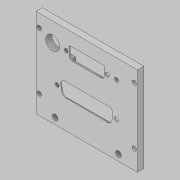
# Autodesk Inventor part: Rückwand_DVI
Saved by Autodesk Inventor 2021.4 (Build 254397000, 397)
## iProperties
Created: 2019-10-17
Part Number: Rückwand_DVI
Material: Generisch
Document SubType Name: Modeling
Designer: Scope
Density: 1 g/cm^3
Appearance: Vorgabe
Author: Scope
Autodesk Inventor part; units mm, degrees
ref_plane "YZ Plane" through (0, 0, 0) normal (1, 0, 0) x (0, 1, 0)
ref_plane "XZ Plane" through (0, 0, 0) normal (0, 1, 0) x (-1, 0, 0)
ref_plane "XY Plane" through (0, 0, 0) normal (0, 0, 1) x (1, 0, 0)
sketch "Skizze1" plane through (0, 0, 0) normal (0, 0, 1) x (1, 0, 0)
  line L0 (-40, 35) -> (40, 35)
  line L1 (40, 35) -> (40, -35)
  line L2 (40, -35) -> (-40, -35)
  line L3 (-40, -35) -> (-40, 35)
  line L4 (-40, 35) -> (40, -35) construction
  line L5 (40, 35) -> (-40, -35) construction
  point P0 (0, 0)
  dimension "d0" = 80
  dimension "d1" = 70
  constraints: 12 end point, 2 midpoint, 2 parallel, 1 horizontal, 1 perpendicular
  measures "d0" distance between parallel lines of L1 L3
  measures "d1" distance between parallel lines of L2 L0
extrude "Extrusion1" add sketch "Skizze1" along normal blind 5
sketch "Skizze2" plane through (0, 0, 5) normal (0, 0, 1) x (1, 0, 0)
  line L0 (-37.5, 25) -> (37.5, 25)
  line L1 (37.5, 25) -> (37.5, -20)
  line L2 (37.5, -20) -> (-37.5, -20)
  line L3 (-37.5, -20) -> (-37.5, 25)
  line L4 (-40, 35) -> (-40, -35) projected
  line L5 (40, -35) -> (40, 35) projected
  line L6 (-40, -35) -> (40, -35) projected
  point P0 (0, 0)
  dimension "d4" = 2.5
  dimension "d5" = 2.5
  dimension "d6" = 15
  dimension "d7" = 60
  constraints: 8 end point, 2 parallel, 1 horizontal, 1 perpendicular
  measures "d4" distance between parallel lines of L3 L4
  measures "d5" distance between parallel lines of L5 L1
  measures "d6" distance between parallel lines of L2 L6
  measures "d7" distance between parallel lines of L0 L6
hole "Bohrung1" at (-37.5, 25, 5) at (37.5, 25, 5) at (37.5, -20, 5) at (-37.5, -20, 5) direction (0, 0, -1) diameter 3.4 end through all clearance for "Flachkopfmaschinenschraube" size "M3" standard "ANSI Metrisches M Profil"
sketch "Skizze3" plane through (0, 0, 5) normal (0, 0, 1) x (1, 0, 0)
  line L0 (-25, -30) -> (25, -30)
  line L1 (-40, 35) -> (-40, -35) projected
  line L2 (40, -35) -> (40, 35) projected
  line L3 (-40, -35) -> (40, -35) projected
  point P0 (0, 0)
  dimension "d15" = 15
  dimension "d16" = 15
  dimension "d17" = 5
  constraints: 2 end point, 1 horizontal
  measures "d15" distance from line of L1 L0.start
  measures "d16" distance from line of L0.end L2
  measures "d17" distance between parallel lines of L3 L0
hole "Bohrung2" at (-25, -30, 5) at (25, -30, 5) direction (0, 0, -1) diameter 4.5 end through all clearance for "Flachkopfmaschinenschraube" size "M4" standard "ANSI Metrisches M Profil"
sketch "Skizze4" plane through (0, 0, 5) normal (0, 0, 1) x (1, 0, 0)
  line L0 (-13.15, 24.8) -> (13.15, 24.8)
  line L1 (13.75, 24.2) -> (13.75, 17.7)
  line L2 (11.25, 15.2) -> (-11.25, 15.2)
  line L3 (-13.75, 17.7) -> (-13.75, 24.2)
  line L4 (-13.75, 24.8) -> (13.75, 15.2) construction
  line L5 (13.75, 24.8) -> (-13.75, 15.2) construction
  line L6 (40, 35) -> (-40, 35) projected
  arc A0 (-13.15, 24.8) -> (-13.75, 24.2) centre (-13.15, 24.2) ccw
  arc A1 (13.75, 24.2) -> (13.15, 24.8) centre (13.15, 24.2) ccw
  arc A2 (-13.75, 17.7) -> (-11.25, 15.2) centre (-11.25, 17.7) ccw
  arc A3 (11.25, 15.2) -> (13.75, 17.7) centre (11.25, 17.7) ccw
  line L7 (48.751, 18.7264) -> (89.4803, 18.7264) construction
  line L8 (89.4803, 18.7264) -> (89.4803, 14.9967) construction
  line L9 (89.4803, 14.9967) -> (48.751, 14.9967) construction
  line L10 (48.751, 14.9967) -> (48.751, 18.7264) construction
  line L11 (-17.198, -1.3) -> (17.198, -1.3)
  line L12 (21.25, -1.3) -> (21.25, -1.3)
  line L13 (16.3869, -12.7) -> (-16.3869, -12.7)
  line L14 (-21.25, -1.3) -> (-21.25, -1.3)
  line L15 (-21.25, -1.3) -> (21.25, -12.7) construction
  line L16 (21.25, -1.3) -> (-21.25, -12.7) construction
  line L17 (-40, -35) -> (40, -35) projected
  line L18 (-20.5464, -5.2904) -> (-19.7353, -9.8904)
  line L19 (20.5464, -5.2904) -> (19.7353, -9.8904)
  arc A4 (-17.198, -1.3) -> (-20.5464, -5.2904) centre (-17.198, -4.7) ccw
  arc A5 (20.5464, -5.2904) -> (17.198, -1.3) centre (17.198, -4.7) ccw
  arc A6 (-19.7353, -9.8904) -> (-16.3869, -12.7) centre (-16.3869, -9.3) ccw
  arc A7 (16.3869, -12.7) -> (19.7353, -9.8904) centre (16.3869, -9.3) ccw
  line L20 (50.079, -7.9738) -> (119.9486, -7.9738) construction
  line L21 (119.9486, -7.9738) -> (119.9486, -12.597) construction
  line L22 (119.9486, -12.597) -> (50.079, -12.597) construction
  line L23 (50.079, -12.597) -> (50.079, -7.9738) construction
  line L24 (40, -35) -> (40, 35) projected
  point P0 (0, 0)
  point P1 (0, 20)
  point P2 (0, 20)
  point P3 (0, -7)
  point P4 (0, -7)
  point P5 (0, -7)
  point P6 (-19.2399, -12.7)
  point P7 (19.2399, -12.7)
  dimension "d25" = 27.5
  dimension "d26" = 9.6
  dimension "d28" = 0.6
  dimension "d29" = 2.5
  dimension "d32" = 15
  dimension "d49" = 28
  dimension "d50" = 11.4
  dimension "d51" = 42.5
  dimension "d52" = 80
  dimension "d53" = 19.2399
  dimension "d54" = 19.2399
  dimension "d55" = 80
  dimension "d56" = 3.4
  dimension "d64" = 26.25
  constraints: 28 end point, 20 point on line, 16 point on circle, 16 tangent, 8 centre point, 7 midpoint, 5 equal radius, 4 parallel, 2 horizontal, 2 perpendicular, 2 vertical alignment, 4 other
  measures "d25" distance between parallel lines of L1 L3
  measures "d26" distance of L5.start L4.end
  measures "d28" radius of A0
  measures "d29" radius of A2
  measures "d32" distance from line of L6 point (0, 20)
  measures "d49" distance from line of L17 point (0, -7)
  measures "d50" distance between parallel lines of L13 L11
  measures "d51" distance between parallel lines of L12 L14
  measures "d52" angle of L11 L18
  measures "d53" horizontal distance of point (0, -7) point (-19.24, -12.7)
  measures "d54" horizontal distance of point (19.24, -12.7) point (0, -7)
  measures "d55" angle of L19 L11
  measures "d56" radius of A4
  measures "d64" distance between parallel lines of L1 L24
extrude "Extrusion2" cut sketch "Skizze4" against normal through all
sketch "Skizze5" plane through (0, 0, 5) normal (0, 0, 1) x (1, 0, 0)
  line L0 (40, 35) -> (-40, 35) projected
  line L1 (0, -7) -> (23.5, -7)
  line L2 (0, -7) -> (-23.5, -7)
  line L3 (-40, -35) -> (40, -35) projected
  line L4 (-13.75, 17.7) -> (-13.75, 24.2) projected
  line L5 (13.75, 24.2) -> (13.75, 17.7) projected
  point P0 (0, 0)
  point P1 (-16.25, 20)
  point P2 (16.25, 20)
  dimension "d57" = 28
  dimension "d58" = 23.5
  dimension "d59" = 23.5
  dimension "d65" = 15
  dimension "d66" = 2.5
  dimension "d67" = 2.5
  constraints: 4 end point, 2 horizontal, 1 horizontal alignment
  measures "d57" distance from line of L3 L1.start
  measures "d58" distance of L1.end L1.start
  measures "d59" distance of L2.end L1.start
  measures "d65" distance from line of point (-16.25, 20) L0
  measures "d66" distance from line of point (-16.25, 20) L4
  measures "d67" distance from line of L5 point (16.25, 20)
hole "Bohrung3" at (-23.5, -7, 5) at (23.5, -7, 5) at (-16.25, 20, 5) at (16.25, 20, 5) direction (0, 0, -1) diameter 3.1 end through all
sketch "Skizze6" plane through (0, 0, 0) normal (0, 0, -1) x (-1, 0, 0)
  line L0 (40, 35) -> (-40, 35) projected
  line L1 (-26.4, -0.25) -> (26.4, -0.25)
  line L2 (27, -0.85) -> (27, -13.15)
  line L3 (26.4, -13.75) -> (-26.4, -13.75)
  line L4 (-27, -13.15) -> (-27, -0.85)
  line L5 (-27, -0.25) -> (27, -13.75) construction
  line L6 (27, -0.25) -> (-27, -13.75) construction
  line L7 (-40, -35) -> (40, -35) projected
  arc A0 (-26.4, -0.25) -> (-27, -0.85) centre (-26.4, -0.85) ccw
  arc A1 (27, -0.85) -> (26.4, -0.25) centre (26.4, -0.85) ccw
  arc A2 (26.4, -13.75) -> (27, -13.15) centre (26.4, -13.15) ccw
  arc A3 (-27, -13.15) -> (-26.4, -13.75) centre (-26.4, -13.15) ccw
  circle A4 centre (-16.25, 20) radius 1.55 projected
  line L8 (-16.25, 20) -> (16.6724, 20)
  line L9 (13.15, 24.8) -> (-13.15, 24.8) projected
  line L10 (0, 24.8) -> (0, 15.2)
  line L11 (11.25, 15.2) -> (-11.25, 15.2) projected
  line L12 (-18.4, 25.5) -> (18.4, 25.5)
  line L13 (19, 24.9) -> (19, 15.1)
  line L14 (18.4, 14.5) -> (-18.4, 14.5)
  line L15 (-19, 15.1) -> (-19, 24.9)
  line L16 (-19, 25.5) -> (19, 14.5) construction
  line L17 (19, 25.5) -> (-19, 14.5) construction
  arc A5 (-18.4, 25.5) -> (-19, 24.9) centre (-18.4, 24.9) ccw
  arc A6 (19, 24.9) -> (18.4, 25.5) centre (18.4, 24.9) ccw
  arc A7 (18.4, 14.5) -> (19, 15.1) centre (18.4, 15.1) ccw
  arc A8 (-19, 15.1) -> (-18.4, 14.5) centre (-18.4, 15.1) ccw
  point P0 (0, 0)
  point P1 (0, -7)
  point P2 (0, -7)
  point P3 (0, 20)
  dimension "d60" = 28
  dimension "d61" = 13.5
  dimension "d62" = 54
  dimension "d63" = 0.6
  dimension "d68" = 11
  dimension "d69" = 38
  dimension "d70" = 0.6
  constraints: 28 end point, 16 point on circle, 16 point on line, 16 tangent, 8 centre point, 8 midpoint, 6 equal radius, 4 parallel, 3 horizontal, 2 perpendicular, 1 vertical alignment
  measures "d60" distance from line of point (0, -7) L7
  measures "d61" distance between parallel lines of L3 L1
  measures "d62" distance between parallel lines of L2 L4
  measures "d63" radius of A0
  measures "d68" distance between parallel lines of L14 L12
  measures "d69" distance between parallel lines of L13 L15
  measures "d70" radius of A5
extrude "Extrusion3" cut sketch "Skizze6" against normal blind 4.4
sketch "Skizze7" plane through (0, 0, 0) normal (0, 0, -1) x (-1, 0, 0)
  line L0 (40, -35) -> (40, 35) projected
  line L1 (40, 35) -> (-40, 35) projected
  point P0 (0, 0)
  point P1 (27, 20)
hole "Bohrung4" at (-27, 20, 0) direction (0, 0, 1) diameter 11 end through all
sketch "Skizze10" plane through (0, 0, 0) normal (0, 0, -1) x (-1, 0, 0)
  line L0 (40, 35) -> (-40, 35) projected
  point P0 (0, 0)
  point P1 (-23.5, 20)
  dimension "d84" = 15
  dimension "d85" = 23.5
  measures "d84" distance from line of L0 point (-23.5, 20)
  measures "d85" horizontal distance of point (0, 0) point (-23.5, 20)
hole "Bohrung5" at (23.5, 20, 0) direction (0, 0, 1) diameter 3.1 end through all counterbore diameter 3.5 counterbore depth 2.5
sketch "Skizze11" plane through (0, 0, 0) normal (0, 0, -1) x (-1, 0, 0)
  line L0 (40, -35) -> (40, 35) projected
  line L1 (40, 35) -> (-40, 35) projected
  point P0 (0, 0)
  point P1 (27, 7)
  dimension "d93" = 13
  dimension "d94" = 28
  measures "d93" distance from line of L0 point (27, 7)
  measures "d94" distance from line of L1 point (27, 7)
hole "Bohrung6" at (-27, 7, 0) direction (0, 0, 1) diameter 11 depth 4
sketch "Skizze12" plane through (0, 0, 0) normal (0, 0, -1) x (-1, 0, 0)
  arc A0 (-27, -13.15) -> (-26.4, -13.75) centre (-26.4, -13.15) ccw projected
  line L0 (-27, -13.15) -> (27, -13.15)
  line L1 (27, -13.15) -> (27, -23)
  line L2 (25, -25) -> (-25, -25)
  line L3 (-27, -23) -> (-27, -13.15)
  arc A1 (-27, -23) -> (-25, -25) centre (-25, -23) ccw
  arc A2 (25, -25) -> (27, -23) centre (25, -23) ccw
  line L4 (-40, -35) -> (40, -35) projected
  line L5 (-25, 15.2) -> (13.75, 15.2)
  line L6 (13.75, 15.2) -> (13.75, -3)
  line L7 (11.75, -5) -> (-25, -5)
  line L8 (-27, -3) -> (-27, 13.2)
  arc A3 (-27, -3) -> (-25, -5) centre (-25, -3) ccw
  arc A4 (11.75, -5) -> (13.75, -3) centre (11.75, -3) ccw
  arc A5 (-25, 15.2) -> (-27, 13.2) centre (-25, 13.2) ccw
  circle A6 centre (-16.25, 20) radius 1.55 projected
  point P0 (0, 0)
  point P1 (27, -25)
  point P2 (-27, -0.85)
  point P3 (13.75, 17.7)
  point P4 (-11.25, 15.2)
  dimension "d104" = 2
  dimension "d105" = 10
  dimension "d106" = 2
  dimension "d107" = 2
  dimension "d108" = 25
  constraints: 16 end point, 10 point on circle, 10 tangent, 5 centre point, 4 parallel, 3 vertical alignment, 2 equal radius, 2 horizontal, 2 perpendicular, 2 point on line, 1 horizontal alignment
  measures "d104" radius of A1
  measures "d105" distance between parallel lines of L4 L2
  measures "d106" radius of A3
  measures "d107" radius of A5
  measures "d108" distance from line of L7 A6.centre
extrude "Extrusion4" cut sketch "Skizze12" against normal blind 3 contours L0 L1 A2 L2 A1 L3 | L5 L6 A4 L7 A3 L8 A5
